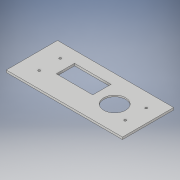
# Autodesk Inventor part: Ausschnitt
Saved by Autodesk Inventor 2017.3 (Build 213256000, 256)
## iProperties
Part Number: Ausschnitt
Material: Generisch
Document SubType Name: Modeling
Designer: Nils
Density: 1 g/cm^3
Appearance: Vorgabe
Author: Nils
Autodesk Inventor part; units mm, degrees
ref_plane "YZ Plane" through (0, 0, 0) normal (1, 0, 0) x (0, 1, 0)
ref_plane "XZ Plane" through (0, 0, 0) normal (0, 1, 0) x (-1, 0, 0)
ref_plane "XY Plane" through (0, 0, 0) normal (0, 0, 1) x (1, 0, 0)
sketch "Skizze1" plane through (0, 0, 0) normal (0, 0, 1) x (1, 0, 0)
  line L0 (25, 12.5) -> (-25, 12.5) projected
  line L1 (-25, 12.5) -> (-25, -12.5) projected
  line L2 (-25, -12.5) -> (25, -12.5) projected
  line L3 (25, -12.5) -> (25, 12.5) projected
  circle A0 centre (50.8, -8.2735) radius 14.6905 projected
  circle A1 centre (50.8, -8.2735) radius 15
  line L4 (-63.7896, 27.9801) -> (95.321, 27.9801)
  line L5 (95.321, 27.9801) -> (95.321, -42.1521)
  line L6 (95.321, -42.1521) -> (-63.7896, -42.1521)
  line L7 (-63.7896, -42.1521) -> (-63.7896, 27.9801)
  point P0 (0, 0)
  dimension "d0" = 30
  constraints: 8 end point, 2 parallel, 1 centre point, 1 coincident, 1 horizontal, 1 perpendicular
  measures "d0" diameter of A1
extrude "Extrusion1" add sketch "Skizze1" along normal blind 3 contours L4 L5 L6 L7
sketch "Skizze2" plane through (0, 0, 0) normal (0, 0, -1) x (-1, 0, 0)
  circle A0 centre (-50.8, -8.2735) radius 15 construction
  circle A1 centre (-50.8, -8.2735) radius 17.5
  point P0 (0, 0)
  dimension "d3" = 35
  constraints: 1 centre point, 1 coincident
  measures "d3" diameter of A1
extrude "Extrusion2" cut sketch "Skizze2" against normal blind 1
sketch "Skizze3" plane through (0, 0, 0) normal (0, 0, -1) x (-1, 0, 0)
  circle A0 centre (-77.33, -20.3235) radius 1.75 construction
  circle A1 centre (40.52, -20.3235) radius 1.75 construction
  circle A2 centre (40.52, 8.5265) radius 1.75 construction
  circle A3 centre (-77.33, 8.5265) radius 1.75 construction
  arc A4 (-44.8513, -25.2196) -> (-44.1338, -24.9216) centre (-45.6338, -22.3235) ccw construction
  arc A5 (-44.8513, -25.2196) -> (-45.0539, -25.3294) centre (-44.7209, -25.7023) ccw construction
  arc A6 (-46.2827, -25.4102) -> (-45.0539, -25.3294) centre (-45.72, -24.5835) ccw construction
  arc A7 (-46.2827, -25.4102) -> (-46.564, -25.3235) centre (-46.564, -25.8235) ccw construction
  line L0 (-55.036, -25.3235) -> (-46.564, -25.3235) construction
  arc A8 (-55.036, -25.3235) -> (-55.3173, -25.4102) centre (-55.036, -25.8235) ccw construction
  arc A9 (-56.4427, -25.4102) -> (-55.3173, -25.4102) centre (-55.88, -24.5835) ccw construction
  arc A10 (-56.4427, -25.4102) -> (-56.724, -25.3235) centre (-56.724, -25.8235) ccw construction
  line L1 (-66.83, -25.3235) -> (-56.724, -25.3235) construction
  arc A11 (-67.83, -24.3235) -> (-66.83, -25.3235) centre (-66.83, -24.3235) ccw construction
  line L2 (-67.83, -14.2262) -> (-67.83, -24.3235) construction
  arc A12 (-67.83, -14.2262) -> (-67.9233, -13.9353) centre (-68.33, -14.2262) ccw construction
  arc A13 (-67.9233, -12.7717) -> (-67.9233, -13.9353) centre (-67.11, -13.3535) ccw construction
  arc A14 (-67.9233, -12.7717) -> (-67.83, -12.4808) centre (-68.33, -12.4808) ccw construction
  line L3 (-67.83, -4.0662) -> (-67.83, -12.4808) construction
  arc A15 (-67.83, -4.0662) -> (-67.9233, -3.7753) centre (-68.33, -4.0662) ccw construction
  arc A16 (-67.9233, -2.6117) -> (-67.9233, -3.7753) centre (-67.11, -3.1935) ccw construction
  arc A17 (-67.9233, -2.6117) -> (-67.83, -2.3208) centre (-68.33, -2.3208) ccw construction
  line L4 (-67.83, -1.6101) -> (-67.83, -2.3208) construction
  arc A18 (-67.83, -1.6101) -> (-68.1376, -1.1483) centre (-68.3305, -1.6101) ccw construction
  arc A19 (-68.445, -0.6869) -> (-68.1376, -1.1483) centre (-67.945, -0.6869) ccw construction
  line L5 (-68.445, 14.5865) -> (-68.445, -0.6869) construction
  arc A20 (-67.945, 15.0865) -> (-68.445, 14.5865) centre (-67.945, 14.5865) ccw construction
  line L6 (-58.801, 15.0865) -> (-67.945, 15.0865) construction
  arc A21 (-58.301, 14.5865) -> (-58.801, 15.0865) centre (-58.801, 14.5865) ccw construction
  line L7 (-58.301, 14.5265) -> (-58.301, 14.5865) construction
  arc A22 (-58.301, 14.5265) -> (-57.301, 13.5265) centre (-57.301, 14.5265) ccw construction
  line L8 (-44.045, 13.5265) -> (-57.301, 13.5265) construction
  arc A23 (-44.045, 13.5265) -> (-43.045, 14.5265) centre (-44.045, 14.5265) ccw construction
  line L9 (-43.045, 14.5865) -> (-43.045, 14.5265) construction
  arc A24 (-42.545, 15.0865) -> (-43.045, 14.5865) centre (-42.545, 14.5865) ccw construction
  line L10 (-33.401, 15.0865) -> (-42.545, 15.0865) construction
  arc A25 (-32.901, 14.5865) -> (-33.401, 15.0865) centre (-33.401, 14.5865) ccw construction
  line L11 (-32.901, 14.5265) -> (-32.901, 14.5865) construction
  arc A26 (-32.901, 14.5265) -> (-31.901, 13.5265) centre (-31.901, 14.5265) ccw construction
  line L12 (21.02, 13.5265) -> (-31.901, 13.5265) construction
  arc A27 (31.02, 3.5265) -> (21.02, 13.5265) centre (21.02, 3.5265) ccw construction
  line L13 (31.02, 2.4539) -> (31.02, 3.5265) construction
  arc A28 (31.02, 2.4539) -> (31.3225, 1.9945) centre (31.52, 2.4539) ccw construction
  arc A29 (31.3225, -0.7615) -> (31.3225, 1.9945) centre (30.73, 0.6165) ccw construction
  arc A30 (31.3225, -0.7615) -> (31.02, -1.2209) centre (31.52, -1.2209) ccw construction
  line L14 (31.02, -1.3561) -> (31.02, -1.2209) construction
  arc A31 (31.02, -1.3561) -> (31.3225, -1.8155) centre (31.52, -1.3561) ccw construction
  arc A32 (31.3225, -4.5715) -> (31.3225, -1.8155) centre (30.73, -3.1935) ccw construction
  arc A33 (31.3225, -4.5715) -> (31.02, -5.0309) centre (31.52, -5.0309) ccw construction
  line L15 (31.02, -5.1661) -> (31.02, -5.0309) construction
  arc A34 (31.02, -5.1661) -> (31.3225, -5.6255) centre (31.52, -5.1661) ccw construction
  arc A35 (31.3225, -8.3815) -> (31.3225, -5.6255) centre (30.73, -7.0035) ccw construction
  arc A36 (31.3225, -8.3815) -> (31.02, -8.8409) centre (31.52, -8.8409) ccw construction
  line L16 (31.02, -10.4303) -> (31.02, -8.8409) construction
  arc A37 (31.02, -10.4303) -> (31.3433, -10.898) centre (31.52, -10.4303) ccw construction
  arc A38 (31.3433, -12.769) -> (31.3433, -10.898) centre (30.99, -11.8335) ccw construction
  arc A39 (31.3433, -12.769) -> (31.02, -13.2367) centre (31.52, -13.2367) ccw construction
  line L17 (31.02, -20.5903) -> (31.02, -13.2367) construction
  arc A40 (31.02, -20.5903) -> (31.3433, -21.058) centre (31.52, -20.5903) ccw construction
  arc A41 (31.3283, -22.9345) -> (31.3433, -21.058) centre (30.99, -21.9935) ccw construction
  arc A42 (31.3283, -22.9345) -> (30.9977, -23.3898) centre (31.4974, -23.4051) ccw construction
  arc A43 (28.77, -25.3235) -> (30.9977, -23.3898) centre (28.77, -23.0735) ccw construction
  line L18 (-24.9736, -25.3235) -> (28.77, -25.3235) construction
  arc A44 (-26.4736, -24.9216) -> (-24.9736, -25.3235) centre (-24.9736, -22.3235) ccw construction
  line L19 (-33.8037, -20.6895) -> (-26.4736, -24.9216) construction
  arc A45 (-33.8037, -20.6895) -> (-36.8037, -20.6895) centre (-35.3037, -23.2876) ccw construction
  line L20 (-44.1338, -24.9216) -> (-36.8037, -20.6895) construction
  line L21 (-81.83, -30.3235) -> (45.02, -30.3235) construction
  arc A46 (45.02, -30.3235) -> (48.02, -27.3235) centre (45.02, -27.3235) ccw construction
  line L22 (48.02, -27.3235) -> (48.02, 15.5265) construction
  arc A47 (48.02, 15.5265) -> (45.02, 18.5265) centre (45.02, 15.5265) ccw construction
  line L23 (45.02, 18.5265) -> (-81.83, 18.5265) construction
  arc A48 (-81.83, 18.5265) -> (-84.83, 15.5265) centre (-81.83, 15.5265) ccw construction
  line L24 (-84.83, 15.5265) -> (-84.83, -27.3235) construction
  arc A49 (-84.83, -27.3235) -> (-81.83, -30.3235) centre (-81.83, -27.3235) ccw construction
  point P0 (0, 0)
  constraints: 4 coincident
hole "Bohrung1" at (77.33, 8.5265, 0) at (77.33, -20.3235, 0) at (-40.52, -20.3235, 0) at (-40.52, 8.5265, 0) direction (0, 0, 1) diameter 3 end through all
